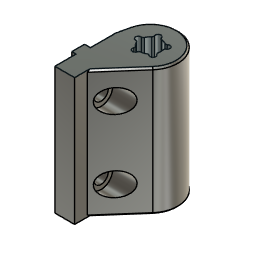
mini_fridge_bottom_latch_left (Autodesk Fusion 360 design; units mm, degrees)
Autodesk Fusion 360 part; units mm, degrees
sketch "Sketch1" plane through (0, 0, 0) normal (0, 0, 1) x (1, 0, 0)
  line L0 (-2.35, 12.52) -> (-7, 12.52)
  line L1 (-7, 12.52) -> (-7, 10.52)
  line L2 (-7, 10.52) -> (-11.5, 10.52)
  line L3 (-11.5, 10.52) -> (-11.5, 7.52)
  line L4 (-11.5, 7.52) -> (-7, 7.52)
  line L5 (-7, 7.52) -> (-7, 1.5)
  line L6 (-2.35, 12.52) -> (4.8823, 4.291)
  line L7 (-7, 1.5) -> (-6.3415, -1.4268)
  arc A0 (-6.3415, -1.4268) -> (4.8823, 4.291) centre (0, 0) ccw
  dimension "d1" = 13
  dimension "d2" = 7
  dimension "d3" = 12.52
  dimension "d4" = 4.65
  dimension "d5" = 2
  dimension "d6" = 4.5
  dimension "d7" = 3
  dimension "d8" = 6.02
  constraint coincident A0.centre origin
  constraint horizontal L0
  constraint perpendicular L0 L1
  constraint perpendicular L1 L2
  constraint perpendicular L2 L3
  constraint perpendicular L3 L4
  constraint perpendicular L4 L5
  constraint tangent L6 A0
  constraint tangent L7 A0
  measures "d1" diameter of A0
  measures "d2" horizontal distance of A0.centre L0.end
  measures "d3" vertical distance of A0.centre L0.end
  measures "d4" distance of L0.start L0.end
  measures "d5" distance of L0.end L1.end
  measures "d6" distance of L1.end L2.end
  measures "d7" distance of L2.end L3.end
  measures "d8" distance of L4.end L5.end
extrude "Extrude1" add sketch "Sketch1" along normal blind 30
sketch "Sketch2" plane through (-11.5, 0, 0) normal (-1, 0, 0) x (0, -1, 0)
  line L0 (-10.52, 0) -> (-7.52, 0)
  line L1 (-7.52, 0) -> (-7.52, 30)
  line L2 (-7.52, 30) -> (-10.52, 30)
  line L3 (-10.52, 30) -> (-10.52, 0)
  circle A0 centre (-9.02, 6.5) radius 2.75
  circle A1 centre (-9.02, 23.5) radius 2.75
  dimension "d11" = 5.5
  dimension "d12" = 5.5
  dimension "d13" = 6.5
  dimension "d14" = 6.5
  measures "d11" diameter of A0
  measures "d12" diameter of A1
  measures "d13" distance of L0 A0.centre
  measures "d14" distance of L2 A1.centre
extrude "Extrude2" cut sketch "Sketch2" against normal blind 27 contours L3 A0 | L1 L3 A0 | L1 A0 | L3 A1 | L1 L3 A1 | L1 A1
sketch "Sketch3" plane through (-11.5, 0, 0) normal (-1, 0, 0) x (0, -1, 0)
  arc A0 (-7.52, 8.8049) -> (-10.52, 8.8049) centre (-9.02, 6.5) ccw
  line L0 (-7.52, 8.8049) -> (-7.52, 21.1951)
  arc A1 (-10.52, 21.1951) -> (-7.52, 21.1951) centre (-9.02, 23.5) ccw
  line L1 (-10.52, 21.1951) -> (-10.52, 8.8049)
  circle A2 centre (-9.02, 23.5) radius 1.7
  circle A3 centre (-9.02, 6.5) radius 1.7
  circle A4 centre (-9.02, 23.5) radius 2.75
  circle A5 centre (-9.02, 6.5) radius 2.75
  dimension "d17" = 3.4
  dimension "d18" = 3.4
  dimension "d19" = 5.5
  dimension "d20" = 5.5
  constraint concentric A1 A2
  constraint concentric A0 A3
  constraint concentric A1 A4
  constraint concentric A3 A5
  measures "d17" diameter of A2
  measures "d18" diameter of A3
  measures "d19" diameter of A4
  measures "d20" diameter of A5
extrude "Extrude3" add sketch "Sketch3" against normal blind 8.9 contours A0 A5 | A1 A4
sketch "Sketch4" plane through (0, 0, 0) normal (0, 0, -1) x (1, 0, 0)
  line L0 (-7, -12.52) -> (-2.35, -12.52)
  line L1 (-2.35, -12.52) -> (4.8823, -4.291)
  arc A0 (4.8823, -4.291) -> (-6.3415, 1.4268) centre (0, 0) ccw
  line L2 (-6.3415, 1.4268) -> (-7, -1.5)
  line L3 (-7, -1.5) -> (-7, -7.52)
  line L4 (-7, -7.52) -> (-11.5, -7.52)
  line L5 (-11.5, -7.52) -> (-11.5, -10.52)
  line L6 (-11.5, -10.52) -> (-7, -10.52)
  line L7 (-7, -10.52) -> (-7, -12.52)
  line L8 (-7, -12.52) -> (-11.5, -12.52)
  line L9 (-11.5, -12.52) -> (-11.5, -10.52)
  line L10 (-11.5, -10.52) -> (-7, -10.52)
  line L11 (-7, -10.52) -> (-7, -12.52)
  line L12 (-7, -7.52) -> (-11.5, -7.52)
  line L13 (-11.5, -7.52) -> (-11.5, -5.1323)
  line L14 (-11.5, -5.1323) -> (-7, -5.1323)
  line L15 (-7, -5.1323) -> (-7, -7.52)
  constraint horizontal L8
  constraint vertical L9
  constraint horizontal L10
  constraint vertical L11
  constraint coincident L5.end L6.start
  constraint coincident L0.start L7.end
  constraint horizontal L12
  constraint vertical L13
  constraint horizontal L14
  constraint vertical L15
  constraint coincident L3.end L4.start
extrude "Extrude4" cut sketch "Sketch4" against normal blind 37 contours L6 L7 L8 L9 L10 L11 | L3 L4 L12 L13 L14 L15
sketch "Sketch5" plane through (0, 12.52, 0) normal (0, 1, 0) x (-1, 0, 0)
  line L0 (2.35, 0) -> (7, 0)
  line L1 (7, 0) -> (7, 30)
  line L2 (7, 30) -> (2.35, 30)
  line L3 (2.35, 30) -> (2.35, 0)
  line L4 (7, 27) -> (13.7208, 27)
  line L5 (13.7208, 27) -> (13.7208, 20)
  line L6 (13.7208, 20) -> (7, 20)
  line L7 (7, 20) -> (7, 27)
  line L8 (7, 10) -> (13.7208, 10)
  line L9 (13.7208, 10) -> (13.7208, 3)
  line L10 (13.7208, 3) -> (7, 3)
  line L11 (7, 3) -> (7, 10)
  line L12 (7, 30) -> (11.5, 30)
  line L13 (7, 0) -> (11.5, 0)
  dimension "d25" = 3
  dimension "d26" = 7
  dimension "d27" = 3
  dimension "d28" = 7
  constraint horizontal L4
  constraint vertical L5
  constraint horizontal L6
  constraint vertical L7
  constraint coincident L1 L4.start
  constraint horizontal L8
  constraint vertical L9
  constraint horizontal L10
  constraint vertical L11
  constraint coincident L1 L8.start
  measures "d25" distance of L4 L12
  measures "d26" distance of L4.end L5.end
  measures "d27" distance of L10 L13
  measures "d28" distance of L8.end L9.end
extrude "Extrude5" cut sketch "Sketch5" against normal blind 27 contours L1 L8 L9 L10 L11 | L1 L4 L5 L6 L7
sketch "Sketch7" plane through (0, 10.52, 0) normal (0, 1, 0) x (-1, 0, 0)
  line L0 (11.5, 20) -> (7, 20)
  line L1 (7, 20) -> (7, 10)
  line L2 (7, 10) -> (11.5, 10)
  line L3 (11.5, 10) -> (11.5, 20)
  line L4 (10, 32.7269) -> (15.8101, 32.7269)
  line L5 (15.8101, 32.7269) -> (15.8101, -2.6481)
  line L6 (15.8101, -2.6481) -> (10, -2.6481)
  line L7 (10, -2.6481) -> (10, 32.7269)
  line L8 (7, 0) -> (7, 30)
  dimension "d31" = 3
  constraint horizontal L4
  constraint vertical L5
  constraint horizontal L6
  constraint vertical L7
  measures "d31" distance of L7 L8
extrude "Extrude6" cut sketch "Sketch7" against normal blind 17 contours L0 L2 L3 L7 | L0 L2 L3 L4 L5 L6 L7
sketch "Sketch8" plane through (0, 0, 0) normal (0, 0, -1) x (1, 0, 0)
  line L0 (-10, -7.52) -> (-10, -10.52)
  line L1 (-10, -10.52) -> (-7, -10.52)
  line L2 (-7, -10.52) -> (-7, -12.52)
  line L3 (-7, -12.52) -> (-2.35, -12.52)
  line L4 (-2.35, -12.52) -> (4.8823, -4.291)
  arc A0 (4.8823, -4.291) -> (-6.3415, 1.4268) centre (0, 0) ccw
  line L5 (-6.3415, 1.4268) -> (-7, -1.5)
  line L6 (-7, -1.5) -> (-7, -7.52)
  line L7 (-7, -7.52) -> (-10, -7.52)
  line L8 (-2.4521, -0.534) -> (-2.438, -0.5533)
  line L9 (-1.2796, -2.1477) -> (-1.2655, -2.167)
  arc A1 (-1.257, -2.161) -> (-0.2532, -2.4871) centre (-0.8776, -2.701) ccw
  arc A2 (-2.4437, 0.5277) -> (-2.4437, -0.5277) centre (-2.84, 0) ccw
  arc A3 (-2.4437, -0.5277) -> (-1.257, -2.161) centre (0, 0) ccw
  arc A4 (-0.2532, 2.4871) -> (-1.257, 2.161) centre (-0.8776, 2.701) ccw
  arc A5 (-1.257, 2.161) -> (-2.4437, 0.5277) centre (0, 0) ccw
  arc A6 (2.2872, 1.0094) -> (1.6668, 1.8633) centre (2.2976, 1.6693) ccw
  arc A7 (1.6668, 1.8633) -> (-0.2532, 2.4871) centre (0, 0) ccw
  arc A8 (1.6668, -1.8633) -> (2.2872, -1.0094) centre (2.2976, -1.6693) ccw
  arc A9 (-0.2532, -2.4871) -> (1.6668, -1.8633) centre (0, 0) ccw
  arc A10 (2.2872, -1.0094) -> (2.2872, 1.0094) centre (0, 0) ccw
  dimension "d34" = 5
  dimension "d35" = 2.84
  dimension "d36" = 1.32
  dimension "d37" = 1.32
  dimension "d38" = 1.32
  dimension "d39" = 1.32
  dimension "d40" = 1.32
  constraint coincident A0.centre A3.centre
  constraint coincident L8.end A9
  constraint coincident L9.start A9
  constraint collinear L8 L9
  constraint coincident A1 L9.end
  constraint coincident A2.end A9
  constraint concentric A3 A9
  constraint coincident A2 L8.start
  constraint coincident A4.end A9
  constraint concentric A5 A9
  constraint coincident A6.end A9
  constraint concentric A7 A9
  constraint coincident A8.end A9
  constraint concentric A9 A10
  measures "d34" diameter of A9
  measures "d35" distance of A0.centre A2.centre
  measures "d36" diameter of A4
  measures "d37" diameter of A6
  measures "d38" diameter of A8
  measures "d39" diameter of A1
  measures "d40" diameter of A2
extrude "Extrude7" cut sketch "Sketch8" against normal blind 25 contours A1 A2 A3 A4 A5 A6 A7 A8 A9 A10
fillet "Fillet1" radius 0.4 10 edges at (-0.2532, -2.4871, 12.5) (1.6668, -1.8633, 12.5) (2.2872, -1.0094, 12.5) (2.2872, 1.0094, 12.5) (-1.257, -2.161, 12.5) (-2.4437, -0.5277, 12.5) (-2.4437, 0.5277, 12.5) (-1.257, 2.161, 12.5) (-0.2532, 2.4871, 12.5) (1.6668, 1.8633, 12.5)
extrude "Extrude8" add 1 faces at (-5.45, 12.52, 20) along direction (0, 1, 0) blind 3
chamfer "Chamfer1" distance 0.4 angle 45 7 edges at (-2.35, 14.02, 0) (-4.675, 15.52, 0) (1.2662, 8.4055, 0) (2.9505, -5.7917, 0) (-6.6707, 0.0366, 0) (-7, 4.51, 0) (-7, 13.02, 0)
chamfer "Chamfer2" distance 0.4 angle 45 6 edges at (1.2662, 8.4055, 30) (-6.6707, 0.0366, 30) (2.9505, -5.7917, 30) (-2.35, 14.02, 30) (-7, 13.02, 30) (-7, 4.51, 30)
chamfer "Chamfer3" distance 0.4 angle 45 1 edges at (-4.675, 15.52, 30)
move_body "Align1" bodies 1 to x (1, 0, 0) y (0, 1, 0) z (0, 0, 1) at (0, 0, 0)
move_body "Move1" bodies 1 to x (1, 0, 0) y (0, -1, 0) z (0, 0, -1) at (0, 8.5031, 60)
move_body "Align2" bodies 1 to x (1, 0, 0) y (0, 1, 0) z (0, 0, 1) at (0, 0, -30)
extrude "Extrude9" cut 3 faces at (-10, -0.0169, 28) (-10, -1.0169, 16.6667) (-10, -1.0169, 2) along direction (1, 0, 0) blind 2
chamfer "Chamfer4" distance 1 angle 45 4 edges at (-7, -0.5169, 27) (-7, -0.5169, 10) (-7, -0.5169, 3) (-7, -0.5169, 20)
delete_face "DeleteFace1" 1 faces at (-4.0333, -6.8836, 29.7333)
delete_face "DeleteFace2" 1 faces at (-6.8667, -3.6836, 29.7333)
delete_face "DeleteFace3" 1 faces at (-2.6167, -4.9667, 29.8667)
delete_face "DeleteFace4" 1 faces at (-4.0333, -6.8836, 0.2667)
delete_face "DeleteFace5" 1 faces at (-6.8667, -5.3503, 0.2667)
delete_face "DeleteFace6" 1 faces at (-2.6167, -4.9667, 0.1333)
sketch "Sketch9" plane through (0, 0, 30) normal (0, 0, 1) x (-1, 0, 0)
  line L0 (2.35, 7.0169) -> (2.35, 3.411)
  line L1 (2.35, 3.411) -> (-4.5819, -4.4761)
  arc A0 (-4.5819, -4.4761) -> (5.9512, -9.8421) centre (0, -8.5031) ccw
  line L2 (5.9512, -9.8421) -> (6.6, -6.9586)
  line L3 (6.6, -6.9586) -> (6.6, -0.9831)
  line L4 (6.6, -0.9831) -> (8, -0.9831)
  line L5 (8, -0.9831) -> (8, 2.0169)
  line L6 (8, 2.0169) -> (7, 2.0169)
  line L7 (7, 2.0169) -> (7, 7.0169)
  line L8 (7, 7.0169) -> (2.35, 7.0169)
  arc A1 (-1.8438, -6.3545) -> (-1.3524, -6.4005) centre (-1.5688, -6.0641) ccw
  arc A2 (-0.1417, -6.0071) -> (-1.3524, -6.4005) centre (0, -8.5031) ccw
  arc A3 (-0.1417, -6.0071) -> (0.2288, -5.6811) centre (-0.1644, -5.6077) ccw
  arc A4 (1.4736, -6.0856) -> (0.2288, -5.6811) centre (0.8776, -5.8021) ccw
  arc A5 (1.4736, -6.0856) -> (1.5818, -6.5671) centre (1.8349, -6.2574) ccw
  arc A6 (2.33, -7.597) -> (1.5818, -6.5671) centre (0, -8.5031) ccw
  arc A7 (2.33, -7.597) -> (2.7546, -7.8486) centre (2.7028, -7.452) ccw
  arc A8 (2.7546, -9.1575) -> (2.7546, -7.8486) centre (2.84, -8.5031) ccw
  arc A9 (2.7546, -9.1575) -> (2.33, -9.4092) centre (2.7028, -9.5542) ccw
  arc A10 (1.5818, -10.4391) -> (2.33, -9.4092) centre (0, -8.5031) ccw
  arc A11 (1.5818, -10.4391) -> (1.4736, -10.9206) centre (1.8349, -10.7488) ccw
  arc A12 (0.2288, -11.3251) -> (1.4736, -10.9206) centre (0.8776, -11.2041) ccw
  arc A13 (0.2288, -11.3251) -> (-0.1417, -10.9991) centre (-0.1644, -11.3984) ccw
  arc A14 (-1.3524, -10.6057) -> (-0.1417, -10.9991) centre (0, -8.5031) ccw
  arc A15 (-1.3524, -10.6057) -> (-1.8438, -10.6516) centre (-1.5688, -10.9421) ccw
  arc A16 (-2.6132, -9.5927) -> (-1.8438, -10.6516) centre (-2.2976, -10.1724) ccw
  arc A17 (-2.6132, -9.5927) -> (-2.4176, -9.1396) centre (-2.8044, -9.2414) ccw
  arc A18 (-2.4176, -7.8666) -> (-2.4176, -9.1396) centre (0, -8.5031) ccw
  arc A19 (-2.4176, -7.8666) -> (-2.6132, -7.4134) centre (-2.8044, -7.7648) ccw
  arc A20 (-1.8438, -6.3545) -> (-2.6132, -7.4134) centre (-2.2976, -6.8338) ccw
